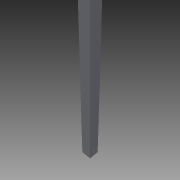
# Autodesk Inventor part: Kick
Saved by Autodesk Inventor 2015 (Build 190159000, 159)
## iProperties
Created: 2018-12-29
Part Number: Kick
Material: Типовые
Document SubType Name: Modeling
Designer: kostya
Density: 1 g/cm^3
Appearance: По умолчанию
Author: kostya
Autodesk Inventor part; units mm, degrees
ref_plane "YZ Plane" through (0, 0, 0) normal (1, 0, 0) x (0, 1, 0)
ref_plane "XZ Plane" through (0, 0, 0) normal (0, 1, 0) x (-1, 0, 0)
ref_plane "XY Plane" through (0, 0, 0) normal (0, 0, 1) x (1, 0, 0)
sketch "Эскиз2" plane through (0, 0, 0) normal (0, 0, 1) x (1, 0, 0)
  line L0 (-5, -5) -> (5, -5)
  line L1 (5, -5) -> (5, 5)
  line L2 (5, 5) -> (-5, 5)
  line L3 (-5, 5) -> (-5, -5)
  line L4 (-5, -5) -> (5, 5) construction
  line L5 (5, -5) -> (-5, 5) construction
  point P0 (0, 0)
  dimension "d4" = 10
  dimension "d5" = 10
  constraints: 12 end point, 2 midpoint, 2 parallel, 1 horizontal, 1 perpendicular
  measures "d4" distance of L2.end L1.end
  measures "d5" distance of L1.end L0.end
extrude "Выдавливание2" add sketch "Эскиз2" along normal blind 155
sketch "Эскиз3" plane through (-5, -5, 0) normal (-1, 0, 0) x (0, 0, 1)
  line L0 (0, 10) -> (0, 0) projected
  line L1 (0, 0) -> (155, 0) projected
  line L2 (155, 10) -> (155, 0) projected
  line L3 (0, 10) -> (155, 10) projected
  line L4 (0, 5) -> (1, 5) construction
  line L5 (1, 5) -> (2, 5) construction
  circle A0 centre (1.5, 5) radius 0.5
  line L6 (2, 5) -> (4, 5) construction
  circle A1 centre (4.5, 5) radius 0.5
  circle A2 centre (7.5, 5) radius 0.5
  point P0 (7, 5)
  dimension "d8" = 1
  dimension "d9" = 1
  dimension "d12" = 2
  dimension "d15" = 3
  constraints: 6 end point, 6 horizontal, 3 horizontal alignment, 1 midpoint, 10 other
  measures "d8" distance of L4.start L4.end
  measures "d9" distance of L4.end L5.end
  measures "d12" distance of L5.end L6.end
  measures "d15" distance of point (1.5, 5) point (4.5, 5)
extrude "Выдавливание3" cut sketch "Эскиз3" against normal blind 155 contours A0 | A1 | A2
sketch "Эскиз4" plane through (0, 0, 155) normal (0, 0, 1) x (1, 0, 0)
  line L0 (-5, -5) -> (5, -5) projected
  line L1 (5, -5) -> (5, 5) projected
  line L2 (5, 5) -> (-5, 5) projected
  line L3 (-5, 5) -> (-5, -5) projected
  point P0 (0, 0)
extrude "Выдавливание4" cut sketch "Эскиз4" against normal blind 15
sketch "Эскиз5" plane through (0, 0, 140) normal (0, 0, 1) x (1, 0, 0)
  circle A0 centre (0, 0) radius 2
  dimension "d22" = 4
  constraints: 1 centre point, 1 coincident
  measures "d22" diameter of A0
extrude "Выдавливание5" cut sketch "Эскиз5" against normal blind 5
